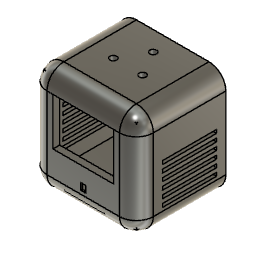
Cube (Autodesk Fusion 360 design; units mm, degrees)
Autodesk Fusion 360 part; units mm, degrees
note: some values were not read from the file. Set by a fixed rule: which face or edge a step refers to.
sketch "Sketch1" plane through (0, 0, 0) normal (0, 0, 1) x (1, 0, 0)
  line L0 (0, 0) -> (80, 0)
  line L1 (80, 0) -> (80, 80)
  line L2 (80, 80) -> (0, 80)
  line L3 (0, 80) -> (0, 0)
  dimension "d1" = 80
  dimension "d2" = 80
  constraint horizontal L0
  constraint vertical L1
  constraint horizontal L2
  constraint vertical L3
  constraint coincident L0.start L3.end
  measures "d1" distance of L0.start L0.end
  measures "d2" distance of L0.start L2.end
extrude "Extrude1" add sketch "Sketch1" along normal blind 80
sketch "Sketch2" plane through (0, 0, 0) normal (0, -1, 0) x (1, 0, 0)
  line L0 (0, 0) -> (80, 0)
  line L1 (80, 0) -> (80, 80)
  line L2 (80, 80) -> (0, 80)
  line L3 (0, 80) -> (0, 0)
  circle A0 centre (40, 40) radius 4.9498
  dimension "d5" = 9.8996
  measures "d5" diameter of A0
shell "Shell1" thickness 5.08 removed faces 1 at (53.3333, 80, 26.6667)
sketch "Sketch4" plane through (0, 0, 0) normal (0, 0, -1) x (1, 0, 0)
  line L0 (0, 0) -> (0, -80)
  line L1 (0, -80) -> (80, -80)
  line L2 (80, -80) -> (80, 0)
  line L3 (80, 0) -> (0, 0)
  circle A0 centre (40, -40) radius 3.65
  dimension "d10" = 7.3
  measures "d10" diameter of A0
extrude "Extrude3" cut sketch "Sketch4" against normal up to surface (5.08 mm away) contours A0
sketch "Sketch5" plane through (0, 0, 80) normal (0, 0, 1) x (-1, 0, 0)
  line L0 (0, -80) -> (0, 0)
  line L1 (0, 0) -> (-80, 0)
  line L2 (-80, 0) -> (-80, -80)
  line L3 (-80, -80) -> (0, -80)
  circle A0 centre (-40, -40) radius 12.7
  circle A1 centre (-40, -52.7) radius 2.54
  circle A2 centre (-29.0015, -33.65) radius 2.54
  circle A3 centre (-50.9985, -33.65) radius 2.54
  dimension "d13" = 25.4
  dimension "d14" = 5.08
  dimension "d16" = 360
  constraint coincident A0 A1.centre
  measures "d13" diameter of A0
  measures "d14" diameter of A1
extrude "Extrude4" cut sketch "Sketch5" against normal up to surface (5.08 mm away) contours A0 A2 | A0 A2 | A0 A1 | A0 A1 | A0 A3 | A0 A3
sketch "Sketch8" plane through (0, 0, 0) normal (0, -1, 0) x (1, 0, 0)
  line L0 (0, 0) -> (80, 0)
  line L1 (80, 0) -> (80, 80)
  line L2 (80, 80) -> (0, 80)
  line L3 (0, 80) -> (0, 0)
  line L4 (17.14, 67.3) -> (62.86, 67.3)
  line L5 (62.86, 67.3) -> (62.86, 31.74)
  line L6 (62.86, 31.74) -> (17.14, 31.74)
  line L7 (17.14, 31.74) -> (17.14, 67.3)
  line L8 (41.905, 20.32) -> (38.095, 20.32)
  line L9 (38.095, 20.32) -> (38.095, 15.24)
  line L10 (38.095, 15.24) -> (41.905, 15.24)
  line L11 (41.905, 15.24) -> (41.905, 20.32)
  line L12 (41.905, 20.32) -> (38.095, 15.24) construction
  line L13 (38.095, 20.32) -> (41.905, 15.24) construction
  line L14 (5.08, 5.08) -> (74.92, 5.08)
  point P0 (40, 17.78)
  dimension "d38" = 45.72
  dimension "d39" = 35.56
  dimension "d40" = 3.81
  dimension "d41" = 5.08
  dimension "d42" = 10.16
  dimension "d43" = 40
  dimension "d44" = 17.14
  dimension "d45" = 12.7
  constraint horizontal L4
  constraint vertical L5
  constraint horizontal L6
  constraint vertical L7
  constraint horizontal L8
  constraint perpendicular L8 L9
  constraint parallel L8 L10
  constraint parallel L9 L11
  constraint coincident L12 P0
  constraint coincident L13 P0
  measures "d38" distance of L4.start L4.end
  measures "d39" distance of L4.start L6.end
  measures "d40" distance of L9.end L10.end
  measures "d41" distance of L8.end L9.end
  measures "d42" distance of L10 L14
  measures "d43" distance of L1 P0
  measures "d44" distance of L1 L5
  measures "d45" distance of L2 L4
extrude "Extrude7" cut sketch "Sketch8" against normal up to surface (5.08 mm away) contours L4 L5 L6 L7 | L8 L9 L10 L11
sketch "Sketch9" plane through (80, 0, 0) normal (1, 0, 0) x (0, 1, 0)
  line L0 (0, 0) -> (80, 0)
  line L1 (80, 0) -> (80, 80)
  line L2 (80, 80) -> (0, 80)
  line L3 (0, 80) -> (0, 0)
  line L4 (19.68, 17.78) -> (60.32, 17.78)
  line L5 (60.32, 17.78) -> (60.32, 15.24)
  line L6 (60.32, 15.24) -> (19.68, 15.24)
  line L7 (19.68, 15.24) -> (19.68, 17.78)
  line L8 (60.32, 23.368) -> (60.32, 20.828)
  line L9 (19.68, 23.368) -> (60.32, 23.368)
  line L10 (19.68, 20.828) -> (19.68, 23.368)
  line L11 (60.32, 20.828) -> (19.68, 20.828)
  line L12 (60.32, 28.956) -> (60.32, 26.416)
  line L13 (19.68, 28.956) -> (60.32, 28.956)
  line L14 (19.68, 26.416) -> (19.68, 28.956)
  line L15 (60.32, 26.416) -> (19.68, 26.416)
  line L16 (60.32, 34.544) -> (60.32, 32.004)
  line L17 (19.68, 34.544) -> (60.32, 34.544)
  line L18 (19.68, 32.004) -> (19.68, 34.544)
  line L19 (60.32, 32.004) -> (19.68, 32.004)
  line L20 (60.32, 40.132) -> (60.32, 37.592)
  line L21 (19.68, 40.132) -> (60.32, 40.132)
  line L22 (19.68, 37.592) -> (19.68, 40.132)
  line L23 (60.32, 37.592) -> (19.68, 37.592)
  line L24 (60.32, 45.72) -> (60.32, 43.18)
  line L25 (19.68, 45.72) -> (60.32, 45.72)
  line L26 (19.68, 43.18) -> (19.68, 45.72)
  line L27 (60.32, 43.18) -> (19.68, 43.18)
  dimension "d48" = 40.64
  dimension "d50" = 19.68
  dimension "d51" = 15.24
  dimension "d55" = 2.54
  dimension "d58" = 0
  dimension "d59" = 27.94
  constraint horizontal L4
  constraint vertical L5
  constraint horizontal L6
  constraint vertical L7
  measures "d48" distance of L4.start L4.end
  measures "d50" distance of L1 L5
  measures "d51" distance of L0 L6
  measures "d55" distance of L4.start L6.end
extrude "Extrude8" cut sketch "Sketch9" against normal blind 88.9 contours L4 L5 L6 L7
extrude "Extrude9" cut sketch "Sketch9" against normal blind 86.36 contours L8 L9 L10 L11 | L12 L13 L14 L15 | L16 L17 L18 L19 | L20 L21 L22 L23 | L24 L25 L26 L27
sketch "Sketch10" plane through (0, 80, 0) normal (0, 1, 0) x (-1, 0, 0)
  line L0 (-80, 80) -> (-80, 0)
  line L1 (-80, 0) -> (0, 0)
  line L2 (0, 0) -> (0, 80)
  line L3 (-5.08, 74.92) -> (-5.08, 5.08)
  line L4 (-5.08, 5.08) -> (-74.92, 5.08)
  line L5 (-74.92, 5.08) -> (-74.92, 74.92)
  line L6 (-74.92, 74.92) -> (-5.08, 74.92)
  line L7 (0, 80) -> (-80, 80)
  line L8 (-74.92, 74.92) -> (-5.08, 74.92)
  line L9 (-5.08, 74.92) -> (-5.08, 5.08)
  line L10 (-5.08, 5.08) -> (-74.92, 5.08)
  line L11 (-74.92, 5.08) -> (-74.92, 74.92)
  constraint horizontal L8
  constraint vertical L9
  constraint horizontal L10
  constraint vertical L11
  constraint coincident L3.end L4.start
  constraint coincident L5.end L6.start
extrude "Extrude10" add sketch "Sketch10" against normal blind 5.08 contours L3 L4 L5 L6 L8 L9 L10 L11
fillet "Fillet2" radius 12.7 12 edges at (80, 40, 80) (40, 80, 80) (80, 80, 40) (0, 80, 40) (0, 40, 80) (40, 80, 0) (80, 40, 0) (80, 0, 40) (0, 40, 0) (40, 0, 0) (0, 0, 40) (40, 0, 80)
sketch "Sketch13" plane through (0, 80, 0) normal (0, 1, 0) x (-1, 0, 0)
  line L0 (-67.3, 67.3) -> (-67.3, 12.7)
  line L1 (-67.3, 12.7) -> (-12.7, 12.7)
  line L2 (-12.7, 12.7) -> (-12.7, 67.3)
  line L3 (-12.7, 67.3) -> (-67.3, 67.3)
  line L4 (-88.9, 88.9) -> (12.7, 88.9)
  line L5 (12.7, 88.9) -> (12.7, -12.7)
  line L6 (12.7, -12.7) -> (-88.9, -12.7)
  line L7 (-88.9, -12.7) -> (-88.9, 88.9)
  constraint horizontal L4
  constraint vertical L5
  constraint horizontal L6
  constraint vertical L7
extrude "Extrude12" cut sketch "Sketch13" against normal blind 12.7 contours L0 L1 L2 L3 | L4 L5 L6 L7
sketch "Sketch14" plane through (0, 5.08, 0) normal (0, 1, 0) x (-1, 0, 0)
  line L0 (-17.14, 67.3) -> (-17.14, 31.74)
  line L1 (-17.14, 31.74) -> (-62.86, 31.74)
  line L2 (-62.86, 31.74) -> (-62.86, 67.3)
  line L3 (-62.86, 67.3) -> (-17.14, 67.3)
  line L4 (-38.095, 15.24) -> (-41.905, 15.24)
  line L5 (-41.905, 15.24) -> (-41.905, 20.32)
  line L6 (-41.905, 20.32) -> (-38.095, 20.32)
  line L7 (-38.095, 20.32) -> (-38.095, 15.24)
  line L8 (-74.92, 5.08) -> (-5.08, 5.08)
  line L9 (-5.08, 5.08) -> (-5.08, 74.92)
  line L10 (-5.08, 74.92) -> (-74.92, 74.92)
  line L11 (-74.92, 74.92) -> (-74.92, 5.08)
  line L12 (-25, 27.78) -> (-55, 27.78)
  line L13 (-55, 27.78) -> (-55, 7.78)
  line L14 (-55, 7.78) -> (-25, 7.78)
  line L15 (-25, 7.78) -> (-25, 27.78)
  line L16 (-25, 27.78) -> (-55, 7.78) construction
  line L17 (-55, 27.78) -> (-25, 7.78) construction
  point P0 (-40, 17.78)
  dimension "d73" = 30
  dimension "d74" = 20
  constraint horizontal L12
  constraint perpendicular L12 L13
  constraint parallel L12 L14
  constraint parallel L13 L15
  constraint coincident L16 P0
  constraint coincident L17 P0
  measures "d73" distance of L13.end L14.end
  measures "d74" distance of L12.end L13.end
extrude "Extrude13" cut sketch "Sketch14" against normal blind 3.81 contours L12 L13 L14 L15
equation "d5 = 0.374 in + 0.4 mm"
equation "d44 = ( 8 cm - 1.8 in ) / 2"
equation "d50 = ( 8 cm - 1.6 in ) / 2"
